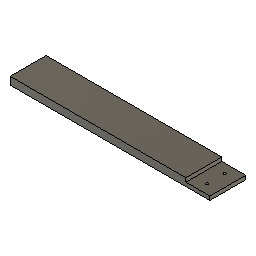
rod1 (Autodesk Fusion 360 design; units mm, degrees)
Autodesk Fusion 360 part; units mm, degrees
sketch "Sketch1" plane through (0, 0, 0) normal (0, 0, 1) x (1, 0, 0)
  line L0 (0, 0) -> (250, 0)
  line L1 (250, 0) -> (250, 45)
  line L2 (250, 45) -> (0, 45)
  line L3 (0, 45) -> (0, 0)
  dimension "d1" = 250
  dimension "d2" = 45
  constraint horizontal L0
  constraint vertical L1
  constraint horizontal L2
  constraint vertical L3
  constraint coincident L0.start L3.end
  measures "d1" distance of L0.start L0.end
  measures "d2" distance of L0.start L2.end
extrude "Extrude1" add sketch "Sketch1" along normal blind 9.5
extrude "Extrude2" add 1 faces at (83.3333, 30, 9.5) along direction (0, 0, 1) blind 0.1
sketch "Sketch2" plane through (0, 0, 9.6) normal (0, 0, 1) x (-1, 0, 0)
  line L0 (0, -45) -> (0, 0)
  line L1 (0, 0) -> (-250, 0)
  line L2 (-250, 0) -> (-250, -45)
  line L3 (-250, -45) -> (0, -45)
  line L4 (-250, -45) -> (-220, -45)
  line L5 (-220, -45) -> (-220, 0)
  line L6 (-220, 0) -> (-250, 0)
  line L7 (-250, 0) -> (-250, -45)
  dimension "d7" = 30
  constraint horizontal L4
  constraint vertical L5
  constraint horizontal L6
  constraint vertical L7
  constraint coincident L2.end L3.start
  measures "d7" distance of L2.end L4.end
extrude "Extrude3" cut sketch "Sketch2" against normal blind 4.8 contours L1 L2 L3 L4 L5 L6 L7
sketch "Sketch3" plane through (0, 0, 4.8) normal (0, 0, 1) x (-1, 0, 0)
  line L0 (-250, 0) -> (-250, -45)
  line L1 (-250, -45) -> (-220, -45)
  line L2 (-220, -45) -> (-220, 0)
  line L3 (-220, 0) -> (-250, 0)
  circle A0 centre (-235, -33.75) radius 1.55
  circle A1 centre (-235, -11.25) radius 1.55
  dimension "d10" = 3.1
  dimension "d11" = 3.1
  measures "d10" diameter of A0
  measures "d11" diameter of A1
extrude "Extrude4" cut sketch "Sketch3" against normal blind 23 contours A0 | A1
equation "d8 = ( -9.6 / 2 ) * 1 mm"
